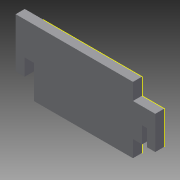
# Autodesk Inventor part: ex_holder_side
Saved by Autodesk Inventor 2014 SP1 (Build 180222100, 222)
## iProperties
Created: 2014-01-31
Part Number: ex_holder_side
Material: Wood (Birch)
Document SubType Name: Modeling
Designer: aoki
Density: 0.55 g/cm^3
Appearance: Birch - Natural Polished
Author: aoki
Autodesk Inventor part; units mm, degrees
ref_plane "YZ Plane" through (0, 0, 0) normal (1, 0, 0) x (0, 1, 0)
ref_plane "XZ Plane" through (0, 0, 0) normal (0, 1, 0) x (-1, 0, 0)
ref_plane "XY Plane" through (0, 0, 0) normal (0, 0, 1) x (1, 0, 0)
sketch "Sketch1" plane through (0, 0, 0) normal (0, 1, 0) x (-1, 0, 0)
  line L0 (30, -20) -> (-30, -20)
  line L1 (-30, -20) -> (-30, 20)
  line L2 (-30, 20) -> (30, 20)
  line L3 (30, 20) -> (30, -20)
  line L4 (30, -20) -> (-30, 20) construction
  line L5 (-30, -20) -> (30, 20) construction
  point P0 (0, 0)
  dimension "d0" = 60
  dimension "d1" = 40
  constraints: 12 end point, 2 midpoint, 2 parallel, 1 horizontal, 1 perpendicular
  measures "d0" distance of L1.end L2.end
  measures "d1" distance of L0.end L1.end
extrude "Extrusion1" add sketch "Sketch1" along normal blind 5.5
sketch "Sketch2" plane through (0, 5.5, 0) normal (0, 1, 0) x (1, 0, 0)
  line L0 (30, -20) -> (30, 20) projected
  line L1 (30, 0) -> (43.5, 0)
  line L2 (43.5, 0) -> (43.5, 10)
  line L3 (43.5, 10) -> (30, 10)
  line L4 (30, 10) -> (30, 0)
  line L5 (-43.1, 0) -> (48.6, 0) projected
  line L6 (43.5, 0) -> (43.5, -10)
  line L7 (43.5, -10) -> (30, -10)
  line L8 (30, -10) -> (30, 0)
  point P0 (0, 0)
  dimension "d4" = 13.5
  dimension "d5" = 10
  constraints: 14 end point, 2 parallel, 2 symmetric about line, 1 horizontal, 1 midpoint, 1 perpendicular
  measures "d4" distance of L3.end L2.end
  measures "d5" distance of L2.end L1.end
extrude "Extrusion2" add sketch "Sketch2" against normal blind 5.5
sketch "Sketch3" plane through (0, 5.5, 0) normal (0, 1, 0) x (1, 0, 0)
  line L0 (43.5, 10) -> (30, 10) projected
  line L1 (30, 10) -> (30, 20) projected
  line L2 (35.5, 10) -> (38.5, 10)
  line L3 (38.5, 10) -> (38.5, 0)
  line L4 (38.5, 0) -> (35.5, 0)
  line L5 (35.5, 0) -> (35.5, 10)
  point P0 (0, 0)
  dimension "d8" = 5.5
  dimension "d9" = 3
  dimension "d10" = 10
  constraints: 8 end point, 2 parallel, 1 horizontal, 1 perpendicular, 1 point on line
  measures "d8" distance between parallel lines of L5 L1
  measures "d9" distance of L3.end L4.end
  measures "d10" distance of L2.end L3.end
extrude "Extrusion3" cut sketch "Sketch3" against normal through all
sketch "Sketch4" plane through (0, 5.5, 0) normal (0, 1, 0) x (1, 0, 0)
  line L0 (35.5, 0) -> (35.5, 10) projected
  line L1 (35.5, 10) -> (30, 10) projected
  line L2 (30, 10) -> (30, 20) projected
  line L3 (30, 20) -> (-30, 20) projected
  line L4 (-30, 20) -> (-30, -20) projected
  line L5 (-30, -20) -> (30, -20) projected
  line L6 (30, -20) -> (30, -10) projected
  line L7 (30, -10) -> (43.5, -10) projected
  line L8 (43.5, -10) -> (43.5, 10) projected
  line L9 (43.5, 10) -> (38.5, 10) projected
  line L10 (38.5, 10) -> (38.5, 0) projected
  line L11 (38.5, 0) -> (35.5, 0) projected
  point P0 (0, 0)
sketch "Sketch5" plane through (0, 5.5, 0) normal (0, 1, 0) x (1, 0, 0)
  line L0 (-30, 20) -> (-30, -20) projected
  line L1 (-44.7, 0) -> (58.2, 0) projected
  line L2 (0, 28) -> (0, -28) projected
  line L3 (-30, 0) -> (-41, 0)
  line L4 (-41, 0) -> (-41, 10)
  line L5 (-41, 10) -> (-30, 10)
  line L6 (-30, 10) -> (-30, 0)
  line L7 (-30, 0) -> (-41, 0)
  line L8 (-41, 0) -> (-41, -20)
  line L9 (-41, -20) -> (-30, -20)
  line L10 (-30, -20) -> (-30, 0)
  point P0 (0, 0)
  dimension "d14" = 11
  dimension "d15" = 10
  constraints: 16 end point, 4 parallel, 2 horizontal, 2 perpendicular, 1 midpoint, 1 point on line
  measures "d14" distance of L4.end L5.end
  measures "d15" distance of L3.end L4.end
extrude "Extrusion4" add sketch "Sketch5" against normal blind 5.5
sketch "Sketch6" plane through (0, 5.5, 0) normal (0, 1, 0) x (1, 0, 0)
  line L0 (-30, 20) -> (-30, 10) projected
  line L1 (-30, 10) -> (-41, 10) projected
  line L2 (-30, 0) -> (-35.5, 0)
  line L3 (-35.5, 0) -> (-35.5, 10)
  line L4 (-35.5, 10) -> (-30, 10)
  line L5 (-30, 10) -> (-30, 0)
  line L6 (-57.9, 0) -> (60.4, 0) projected
  line L7 (0, 28) -> (0, -28) projected
  point P0 (0, 0)
  dimension "d20" = 0
  dimension "d21" = 5.5
  constraints: 8 end point, 2 parallel, 1 horizontal, 1 midpoint, 1 perpendicular
  measures "d20" distance between parallel lines of L0 L5
  measures "d21" distance of L3.end L4.end
extrude "Extrusion5" cut sketch "Sketch6" against normal through all
equation "\"d2\" = Wt"
equation "\"d6\" = Wt"
equation "\"d8\" = Wt"
equation "\"d11\" = Wt"
equation "\"d14\" = 2 * Wt"
equation "\"d16\" = Wt"
equation "\"d21\" = Wt"
equation "\"d22\" = Wt"
equation "\"Wt\" = 5.5"
body "Solid1"
